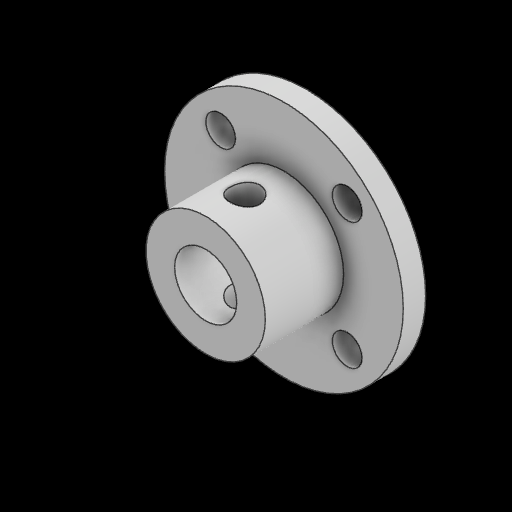
# Autodesk Inventor part: Hub8mm
Saved by Autodesk Inventor 2025.2 (Build 292293000, 293)
## iProperties
Created: 2025-09-16
Part Number: Hub8mm
Material: Generic
Document SubType Name: Modeling
Designer: valer
Density: 1 g/cm^3
Appearance: Default
Author: valer
Autodesk Inventor part; units mm, degrees
ref_plane "YZ Plane" through (0, 0, 0) normal (1, 0, 0) x (0, 1, 0)
ref_plane "XZ Plane" through (0, 0, 0) normal (0, 1, 0) x (-1, 0, 0)
ref_plane "XY Plane" through (0, 0, 0) normal (0, 0, 1) x (1, 0, 0)
sketch "Base" plane through (0, 0, 0) normal (0, 0, 1) x (1, 0, 0)
  circle A0 centre (0, 0) radius 4.165
  circle A1 centre (0, 0) radius 8
  circle A2 centre (0, 0) radius 16
  line L0 (-8.4853, 8.4853) -> (8.4853, 8.4853) construction
  line L1 (8.4853, 8.4853) -> (8.4853, -8.4853) construction
  line L2 (8.4853, -8.4853) -> (-8.4853, -8.4853) construction
  line L3 (-8.4853, -8.4853) -> (-8.4853, 8.4853) construction
  circle A3 centre (0, 0) radius 13.4763 construction
  circle A4 centre (0, 0) radius 14 construction
  circle A5 centre (8.4853, 8.4853) radius 2
  circle A6 centre (8.4853, -8.4853) radius 2
  circle A7 centre (-8.4853, -8.4853) radius 2
  circle A8 centre (-8.4853, 8.4853) radius 2
  dimension "d0" = 8.33
  dimension "d1" = 16
  dimension "d2" = 32
  dimension "d3" = 2.5237
  dimension "d4" = 2
  dimension "d5" = 4
  constraints: 9 centre point, 9 coincident, 8 end point, 3 equal radius, 3 tangent, 2 parallel, 2 perpendicular, 1 horizontal
  measures "d0" diameter of A0
  measures "d1" diameter of A1
  measures "d2" diameter of A2
  measures "d3" radial gap between concentric circles of A2 A3
  measures "d4" radial gap between concentric circles of A2 A4
  measures "d5" diameter of A5
extrude "BaseFeature" add sketch "Base" against normal blind 3 contours A1 | A2
extrude "MountFeature" add sketch "Base" along normal blind 10.5 contours A1
sketch "SetScrewHole" plane through (0, 0, 0) normal (0, 1, 0) x (-1, 0, 0)
  circle A0 centre (0, 5.25) radius 2
  line L0 (8, 10.5) -> (-8, 10.5) construction
  line L1 (-8, 0) -> (8, 0) construction
  line L2 (-4.165, 10.5) -> (4.165, 10.5) projected
  line L3 (0, 10.5) -> (0, 0) construction
  dimension "d10" = 4
  constraints: 2 end point, 2 midpoint, 1 centre point, 1 perpendicular
  measures "d10" diameter of A0
extrude "SetScrewHoleFeature" cut sketch "SetScrewHole" along normal through all both and the other way through all
body "Solid1"
